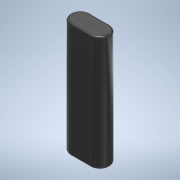
# Autodesk Inventor part: バッテリー
Saved by Autodesk Inventor 2020.2 (Build 242310000, 310)
## iProperties
Part Number: バッテリー
Material: 一般
Document SubType Name: Modeling
Designer: user
Mass: 154 g
Surface Area: 177.801 cm^2
Volume: 127.428 cm^3
Density: 1.20853 g/cm^3
Appearance: 濃い灰色
Author: user
Autodesk Inventor part; units mm, degrees
ref_plane "YZ Plane" through (0, 0, 0) normal (1, 0, 0) x (0, 1, 0)
ref_plane "XZ Plane" through (0, 0, 0) normal (0, 1, 0) x (-1, 0, 0)
ref_plane "XY Plane" through (0, 0, 0) normal (0, 0, 1) x (1, 0, 0)
sketch "スケッチ1" plane through (0, 0, 0) normal (0, 0, 1) x (1, 0, 0)
  line L0 (-11.8937, 2.2764) -> (11.4063, 2.2764) construction
  line L1 (-11.8937, 13.6264) -> (11.4063, 13.6264)
  line L2 (11.4063, -9.0736) -> (-11.8937, -9.0736)
  arc A0 (-11.8937, 13.6264) -> (-11.8937, -9.0736) centre (-11.8937, 2.2764) ccw
  arc A1 (11.4063, -9.0736) -> (11.4063, 13.6264) centre (11.4063, 2.2764) ccw
  point P0 (0, 0)
  point P1 (-0.2437, 2.2764)
  dimension "d0" = 46
  dimension "d1" = 22.7
  constraints: 8 end point, 4 point on circle, 4 tangent, 2 centre point, 1 midpoint, 1 parallel
  measures "d1" distance between parallel lines of L2 L1
extrude "押し出し1" add sketch "スケッチ1" along normal blind 136.7
fillet "フィレット1" radius 2 8 edges at (-0.2437, 13.6264, 136.7) (-23.2437, 2.2764, 136.7) (-0.2437, -9.0736, 136.7) (22.7563, 2.2764, 136.7) (-0.2437, -9.0736, 0) (-23.2437, 2.2764, 0) (-0.2437, 13.6264, 0) (22.7563, 2.2764, 0)
